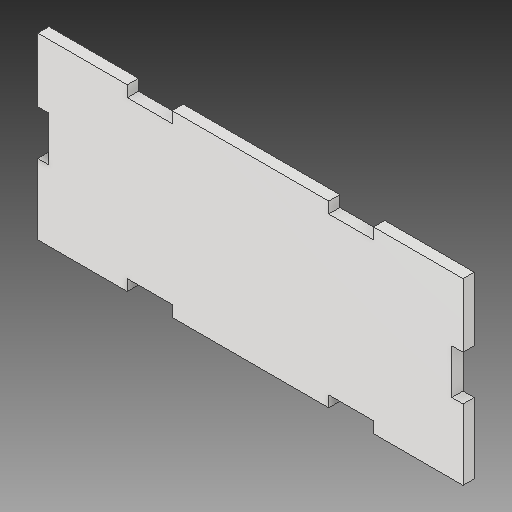
# Autodesk Inventor part: top
Saved by Autodesk Inventor 2018.2 (Build 222227000, 227)
## iProperties
Created: 2018-04-16
Part Number: top
Material: ABS Plastic
Document SubType Name: Modeling
Designer: Derek Fronek
Density: 1.06 g/cm^3
Appearance: Smooth - White
Author: Derek Fronek
Autodesk Inventor part; units mm, degrees
ref_plane "YZ Plane" through (0, 0, 0) normal (1, 0, 0) x (0, 1, 0)
ref_plane "XZ Plane" through (0, 0, 0) normal (0, 1, 0) x (-1, 0, 0)
ref_plane "XY Plane" through (0, 0, 0) normal (0, 0, 1) x (1, 0, 0)
sketch "Sketch1" plane through (0, 0, 0) normal (0, 0, 1) x (1, 0, 0)
  line L0 (117.475, 3.175) -> (117.475, -14.9225) projected
  line L1 (114.3, 3.175) -> (117.475, 3.175) projected
  line L2 (0, -14.9225) -> (-3.175, -14.9225) projected
  line L3 (0, -27.6225) -> (-3.175, -27.6225) projected
  line L4 (0, -14.9225) -> (0, -27.6225)
  line L5 (-3.175, -47.625) -> (-3.175, -27.6225)
  line L6 (-3.175, -14.9225) -> (-3.175, 3.175)
  line L7 (22.225, 0) -> (22.225, 3.175) projected
  line L8 (34.925, 0) -> (34.925, 3.175) projected
  line L9 (34.925, 0) -> (22.225, 0)
  line L10 (-3.175, 3.175) -> (22.225, 3.175)
  line L11 (79.375, 0) -> (79.375, 3.175) projected
  line L12 (92.075, 0) -> (92.075, 3.175) projected
  line L13 (92.075, 0) -> (79.375, 0)
  line L14 (34.925, 3.175) -> (79.375, 3.175)
  line L15 (92.075, 3.175) -> (117.475, 3.175)
  line L16 (114.3, -14.9225) -> (117.475, -14.9225) projected
  line L17 (114.3, -27.6225) -> (117.475, -27.6225) projected
  line L18 (114.3, -14.9225) -> (114.3, -27.6225)
  line L19 (117.475, 3.175) -> (117.475, -14.9225)
  line L20 (117.475, -27.6225) -> (117.475, -47.625)
  line L21 (92.075, -47.625) -> (92.075, -44.45)
  line L22 (92.075, -44.45) -> (79.375, -44.45)
  line L23 (79.375, -44.45) -> (79.375, -47.625)
  line L24 (22.225, -47.625) -> (22.225, -44.45)
  line L25 (22.225, -44.45) -> (34.925, -44.45)
  line L26 (34.925, -44.45) -> (34.925, -47.625)
  line L27 (22.225, -47.625) -> (-3.175, -47.625)
  line L28 (117.475, -47.625) -> (92.075, -47.625)
  line L29 (79.375, -47.625) -> (34.925, -47.625)
  point P0 (0, 0)
  dimension "d0" = 3.175
  constraints: 48 end point, 14 parallel, 9 perpendicular, 5 horizontal, 3 vertical, 2 point on line, 3 other
  measures "d0" distance of L21.start L21.end
extrude "Extrusion1" add sketch "Sketch1" along normal blind 3.175
body "Solid1"
